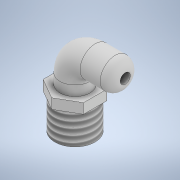
# Autodesk Inventor part: Threaded Elbow
Saved by Autodesk Inventor 2020 (Build 240168000, 168)
## iProperties
Created: 2020-01-14
Part Number: Threaded Elbow
Material: Generic
Document SubType Name: Modeling
Designer: ellio
Density: 1 g/cm^3
Appearance: Default
Author: ellio
Autodesk Inventor part; units mm, degrees
ref_plane "YZ Plane" through (0, 0, 0) normal (1, 0, 0) x (0, 1, 0)
ref_plane "XZ Plane" through (0, 0, 0) normal (0, 1, 0) x (-1, 0, 0)
ref_plane "XY Plane" through (0, 0, 0) normal (0, 0, 1) x (1, 0, 0)
sketch "Sketch1" plane through (0, 0, 0) normal (0, 1, 0) x (-1, 0, 0)
  circle A0 centre (0, 0) radius 6.35
  dimension "d0" = 12.7
  constraints: 1 centre point, 1 coincident
  measures "d0" diameter of A0
extrude "Extrusion1" add sketch "Sketch1" along normal blind 9.525
sketch "Sketch2" plane through (0, 9.525, 0) normal (0, 1, 0) x (1, 0, 0)
  line L0 (0, 7.3892) -> (6.3992, 3.6946)
  line L1 (6.3992, 3.6946) -> (6.3992, -3.6946)
  line L2 (6.3992, -3.6946) -> (0, -7.3892)
  line L3 (0, -7.3892) -> (-6.3992, -3.6946)
  line L4 (-6.3992, -3.6946) -> (-6.3992, 3.6946)
  line L5 (-6.3992, 3.6946) -> (0, 7.3892)
  point P0 (0, 0)
  point P1 (0, 0)
  constraints: 12 end point, 1 coincident, 13 other
extrude "Extrusion2" add sketch "Sketch2" along normal blind 3.175
thread "Thread1" size "1/2-13 UNC" class "2A" standard "ANSI Unified Screw Threads" full length
sketch "Sketch3" plane through (0, 12.7, 0) normal (0, 1, 0) x (1, 0, 0)
  circle A0 centre (0, 0) radius 4.7625
  dimension "d7" = 9.525
  constraints: 1 centre point, 1 coincident
  measures "d7" diameter of A0
extrude "Extrusion3" add sketch "Sketch3" along normal blind 3.175
sketch "Sketch4" plane through (0, 15.875, 0) normal (0, 1, 0) x (1, 0, 0)
  circle A0 centre (0, 0) radius 4.7625
  line L0 (6.3992, -10.3449) -> (6.3992, 10.3449) projected
  constraints: 1 centre point, 1 coincident
revolve "Revolution1" add sketch "Sketch4" angle 90 about axis through (6.3992, 15.875, 3.6946) along (0, 0, -1)
sketch "Sketch5" plane through (6.3992, 22.2742, 0) normal (1, 0, 0) x (0, 0, -1)
  circle A0 centre (0, 0) radius 4.7625 projected
  circle A1 centre (0, 0) radius 4.7625
  point P0 (0, -22.2742)
  constraints: 1 centre point, 1 coincident
extrude "Extrusion4" add sketch "Sketch5" along normal blind 9.525
fillet "Fillet1" radius 3.175 1 edges at (15.9242, 22.2742, 4.7625)
sketch "Sketch6" plane through (15.9242, 22.2742, 0) normal (1, 0, 0) x (0, 0, -1)
  circle A0 centre (0, 0) radius 1.5875
  point P0 (0, -22.2742)
  constraints: 1 centre point
extrude "Extrusion5" cut sketch "Sketch6" against normal blind 9.525
body "Solid1"
